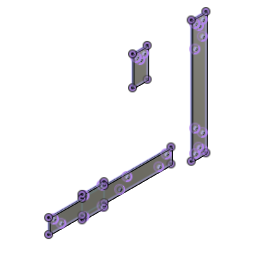
Chassis frame v4 (Autodesk Fusion 360 design; units mm, degrees)
Autodesk Fusion 360 part; units mm, degrees
sketch "Design sketch" plane through (0, 0, 0) normal (1, 0, 0) x (0, 1, 0)
  line L0 (125, 15) -> (-125, 15)
  line L1 (-125, 15) -> (-125, -15)
  line L2 (-125, -15) -> (125, -15)
  line L3 (125, -15) -> (125, 15)
  circle A0 centre (-100, -7.5) radius 1.75
  line L4 (196.3649, 218.9658) -> (166.3649, 218.9658)
  line L5 (166.3649, 218.9658) -> (166.3649, -31.0342)
  line L6 (196.3649, -31.0342) -> (196.3649, 218.9658)
  circle A1 centre (-115, 7.5) radius 1.75
  line L7 (166.3649, -31.0342) -> (196.3649, -31.0342)
  circle A2 centre (100, -7.5) radius 1.75
  circle A3 centre (115, 7.5) radius 1.75
  circle A4 centre (173.8649, 23.9658) radius 1.75
  circle A5 centre (188.8649, 8.9658) radius 1.75
  circle A6 centre (173.8649, 163.9658) radius 1.75
  circle A7 centre (188.8649, 178.9658) radius 1.75
  line L8 (-56.8073, -23.0185) -> (-11.8073, -23.0185)
  line L9 (-11.8073, -23.0185) -> (-11.8073, 21.9815)
  line L10 (-11.8073, 21.9815) -> (-56.8073, 21.9815)
  line L11 (-56.8073, 21.9815) -> (-56.8073, -23.0185)
  circle A8 centre (-52.8073, -19.0185) radius 1.75
  circle A9 centre (-52.8073, 17.9815) radius 1.75
  circle A10 centre (-15.8073, -19.0185) radius 1.75
  circle A11 centre (-15.8073, 17.9815) radius 1.75
  circle A12 centre (35, 7.5) radius 1.75
  circle A13 centre (20, -7.5) radius 1.75
  circle A14 centre (173.8649, -21.0342) radius 1.75
  circle A15 centre (188.8649, -21.0342) radius 1.75
  circle A16 centre (181.3649, -13.5342) radius 1.75
  circle A17 centre (173.8649, 208.9658) radius 1.75
  circle A18 centre (181.3649, 201.4658) radius 1.75
  circle A19 centre (188.8649, 208.9658) radius 1.75
  line L12 (46.3649, 218.9658) -> (76.3649, 218.9658)
  line L13 (76.3649, 218.9658) -> (76.3649, 158.9658)
  line L14 (76.3649, 158.9658) -> (46.3649, 158.9658)
  line L15 (46.3649, 158.9658) -> (46.3649, 218.9658)
  circle A20 centre (53.8649, 208.9658) radius 1.75
  circle A21 centre (61.3649, 201.4658) radius 1.75
  circle A22 centre (68.8649, 208.9658) radius 1.75
  point P0 (20, -7.5)
  dimension "d1" = 250
  dimension "d2" = 30
  dimension "d8" = 3.5
  dimension "d30" = 3.5
  dimension "d49" = 3.5
  dimension "d50" = 3.5
  dimension "d53" = 15
  dimension "d66" = 15
  dimension "d67" = 15
  dimension "d68" = 3.5
  dimension "d69" = 3.5
  dimension "d75" = 15
  dimension "d78" = 30
  dimension "d79" = 250
  dimension "d83" = 15
  dimension "d84" = 15
  dimension "d85" = 3.5
  dimension "d86" = 3.5
  dimension "d87" = 15
  dimension "d89" = 15
  dimension "d92" = 10
  dimension "d93" = 10
  dimension "d94" = 40
  dimension "d95" = 40
  dimension "d96" = 7.5
  dimension "d98" = 7.5
  dimension "d99" = 7.5
  dimension "d100" = 7.5
  dimension "d101" = 45
  dimension "d102" = 45
  dimension "d103" = 3.5
  dimension "d104" = 3.5
  dimension "d105" = 3.5
  dimension "d106" = 3.5
  dimension "d107" = 4
  dimension "d108" = 4
  dimension "d109" = 4
  dimension "d110" = 4
  dimension "d111" = 4
  dimension "d112" = 4
  dimension "d113" = 4
  dimension "d114" = 4
  dimension "d115" = 3.5
  dimension "d116" = 15
  dimension "d117" = 15
  dimension "d118" = 7.5
  dimension "d119" = 3.5
  dimension "d131" = 3.5
  dimension "d132" = 3.5
  dimension "d133" = 15
  dimension "d135" = 3.5
  dimension "d136" = 7.5
  dimension "d137" = 7.5
  dimension "d138" = 10
  dimension "d139" = 3.5
  dimension "d140" = 3.5
  dimension "d141" = 15
  dimension "d142" = 3.5
  dimension "d144" = 7.5
  dimension "d145" = 7.5
  dimension "d146" = 10
  dimension "d147" = 30
  dimension "d148" = 60
  dimension "d149" = 3.5
  dimension "d150" = 3.5
  dimension "d151" = 15
  dimension "d152" = 3.5
  dimension "d153" = 7.5
  dimension "d154" = 7.5
  dimension "d155" = 7.5
  dimension "d156" = 10
  constraint horizontal L0
  constraint perpendicular L0 L1
  constraint parallel L0 L2
  constraint parallel L1 L3
  constraint horizontal L4
  constraint perpendicular L4 L5
  constraint parallel L4 L7
  constraint parallel L5 L6
  constraint horizontal L8
  constraint vertical L9
  constraint horizontal L10
  constraint vertical L11
  constraint coincident P0 A13.centre
  constraint horizontal A14.centre A15.centre
  constraint horizontal A17.centre A19.centre
  constraint horizontal L12
  constraint vertical L13
  constraint horizontal L14
  constraint vertical L15
  constraint horizontal A20.centre A22.centre
  measures "d1" distance of L1.end L2.end
  measures "d2" distance of L0.end L1.end
  measures "d8" diameter of A0
  measures "d30" diameter of A1
  measures "d49" diameter of A2
  measures "d50" diameter of A3
  measures "d53" horizontal distance of A2.centre A3.centre
  measures "d66" vertical distance of A0.centre A1.centre
  measures "d67" horizontal distance of A0.centre A1.centre
  measures "d68" diameter of A4
  measures "d69" diameter of A5
  measures "d75" vertical distance of A2.centre A3.centre
  measures "d78" distance of L5.end L6.start
  measures "d79" distance of L4.start L6.start
  measures "d83" horizontal distance of A4.centre A5.centre
  measures "d84" vertical distance of A4.centre A5.centre
  measures "d85" diameter of A6
  measures "d86" diameter of A7
  measures "d87" horizontal distance of A6.centre A7.centre
  measures "d89" vertical distance of A6.centre A7.centre
  measures "d92" distance of L3 A3.centre
  measures "d93" distance of L1 A1.centre
  measures "d94" distance of L7 A5.centre
  measures "d95" distance of L4 A7.centre
  measures "d96" distance of L2 A2.centre
  measures "d98" distance of L5 A4.centre
  measures "d99" distance of L2 A0.centre
  measures "d100" distance of L5 A6.centre
  measures "d101" distance of L8.start L8.end
  measures "d102" distance of L8.start L10.end
  measures "d103" diameter of A8
  measures "d104" diameter of A9
  measures "d105" diameter of A10
  measures "d106" diameter of A11
  measures "d107" distance of L9 A10.centre
  measures "d108" distance of L8 A10.centre
  measures "d109" distance of L8 A8.centre
  measures "d110" distance of L11 A8.centre
  measures "d111" distance of L10 A9.centre
  measures "d112" distance of L11 A9.centre
  measures "d113" distance of L10 A11.centre
  measures "d114" distance of L9 A11.centre
  measures "d115" diameter of A12
  measures "d116" horizontal distance of P0 A12.centre
  measures "d117" vertical distance of P0 A12.centre
  measures "d118" distance of L2 P0
  measures "d119" diameter of A13
  measures "d131" diameter of A14
  measures "d132" diameter of A15
  measures "d133" horizontal distance of A14.centre A15.centre
  measures "d135" diameter of A16
  measures "d136" vertical distance of A14.centre A16.centre
  measures "d137" horizontal distance of A14.centre A16.centre
  measures "d138" distance of L7 A14.centre
  measures "d139" diameter of A17
  measures "d140" diameter of A19
  measures "d141" horizontal distance of A17.centre A19.centre
  measures "d142" diameter of A18
  measures "d144" horizontal distance of A18.centre A17.centre
  measures "d145" vertical distance of A18.centre A19.centre
  measures "d146" distance of L4 A19.centre
  measures "d147" distance of L12.start L12.end
  measures "d148" distance of L12.end L13.end
  measures "d149" diameter of A20
  measures "d150" diameter of A22
  measures "d151" horizontal distance of A20.centre A22.centre
  measures "d152" diameter of A21
  measures "d153" horizontal distance of A20.centre A21.centre
  measures "d154" vertical distance of A22.centre A21.centre
  measures "d155" distance of L15 A20.centre
  measures "d156" distance of L12 A20.centre
extrude "Extrude6" add sketch "Design sketch" along normal blind 3 makes body 1 at (0, -70.6452, -2.3357) makes body 2 at (0, 61.4084, 172.5507) makes body 3 at (0, 185.1196, 116.9837)
sketch "Sketch7" plane through (0, 0, 0) normal (1, 0, 0) x (0, 0, -1)
  circle A0 centre (-201.4658, 61.3649) radius 1.75
  circle A1 centre (-208.9658, 53.8649) radius 1.75
  circle A2 centre (-208.9658, 68.8649) radius 1.75
  line L0 (-158.9658, 46.3649) -> (-218.9658, 46.3649)
  line L1 (-218.9658, 46.3649) -> (-218.9658, 76.3649)
  line L2 (-218.9658, 76.3649) -> (-158.9658, 76.3649)
  line L3 (-158.9658, 76.3649) -> (-158.9658, 46.3649)
  circle A3 centre (-208.9658, 188.8649) radius 1.75
  circle A4 centre (-201.4658, 181.3649) radius 1.75
  circle A5 centre (-208.9658, 173.8649) radius 1.75
  circle A6 centre (13.5342, 181.3649) radius 1.75
  circle A7 centre (21.0342, 188.8649) radius 1.75
  circle A8 centre (21.0342, 173.8649) radius 1.75
  circle A9 centre (-178.9658, 188.8649) radius 1.75
  circle A10 centre (-8.9658, 188.8649) radius 1.75
  circle A11 centre (-163.9658, 173.8649) radius 1.75
  circle A12 centre (-23.9658, 173.8649) radius 1.75
  line L4 (-218.9658, 166.3649) -> (31.0342, 166.3649)
  line L5 (-218.9658, 196.3649) -> (-218.9658, 166.3649)
  line L6 (31.0342, 196.3649) -> (-218.9658, 196.3649)
  line L7 (31.0342, 166.3649) -> (31.0342, 196.3649)
  circle A13 centre (7.5, 20) radius 1.75
  circle A14 centre (-7.5, 35) radius 1.75
  circle A15 centre (-7.5, -115) radius 1.75
  circle A16 centre (-7.5, 115) radius 1.75
  circle A17 centre (7.5, 100) radius 1.75
  circle A18 centre (-17.9815, -52.8073) radius 1.75
  circle A19 centre (19.0185, -15.8073) radius 1.75
  circle A20 centre (7.5, -100) radius 1.75
  circle A21 centre (-17.9815, -15.8073) radius 1.75
  circle A22 centre (19.0185, -52.8073) radius 1.75
  line L8 (-21.9815, -11.8073) -> (-21.9815, -56.8073)
  line L9 (-15, -11.8073) -> (-21.9815, -11.8073)
  line L10 (-15, 125) -> (-15, -11.8073)
  line L11 (15, 125) -> (-15, 125)
  line L12 (15, -11.8073) -> (15, 125)
  line L13 (23.0185, -11.8073) -> (15, -11.8073)
  line L14 (23.0185, -56.8073) -> (23.0185, -11.8073)
  line L15 (15, -56.8073) -> (23.0185, -56.8073)
  line L16 (15, -125) -> (15, -56.8073)
  line L17 (-15, -125) -> (15, -125)
  line L18 (-15, -56.8073) -> (-15, -125)
  line L19 (-21.9815, -56.8073) -> (-15, -56.8073)
extrude "Extrude2" [suppressed]
equation "d1 = partLength"
equation "d2 = partWidth"
equation "partLength = 250 mm"
equation "partWidth = 30 mm"
equation "boltHole = 3.5 mm"
equation "d8 = boltHole"
equation "boltTriangleHeight = 7 mm"
equation "boltFromEdgesClose = 10 mm"
equation "boltGap = 15 mm"
equation "d30 = boltHole"
equation "boltFromEdgesFar = 40 mm"
equation "d49 = boltHole"
equation "d50 = boltHole"
equation "d53 = boltGap"
equation "d66 = boltGap"
equation "d67 = boltGap"
equation "d68 = boltHole"
equation "d69 = boltHole"
equation "d75 = boltGap"
equation "d78 = partWidth"
equation "d79 = partLength"
equation "d83 = boltGap"
equation "d84 = boltGap"
equation "d85 = boltHole"
equation "d86 = boltHole"
equation "d87 = boltGap"
equation "d89 = boltGap"
equation "d92 = boltFromEdgesClose"
equation "d93 = boltFromEdgesClose"
equation "d94 = boltFromEdgesFar"
equation "d95 = boltFromEdgesFar"
equation "d96 = ( partWidth - boltGap ) / 2"
equation "boltGapFromSide = ( partWidth - boltGap ) / 2"
equation "d98 = boltGapFromSide"
equation "d99 = boltGapFromSide"
equation "d100 = boltGapFromSide"
equation "d107 = ( ( 45 - 37 ) / 2 ) * 1 mm"
equation "d108 = ( ( 45 - 37 ) / 2 ) * 1 mm"
equation "d109 = ( ( 45 - 37 ) / 2 ) * 1 mm"
equation "d110 = ( ( 45 - 37 ) / 2 ) * 1 mm"
equation "d111 = ( ( 45 - 37 ) / 2 ) * 1 mm"
equation "d112 = ( ( 45 - 37 ) / 2 ) * 1 mm"
equation "d113 = ( ( 45 - 37 ) / 2 ) * 1 mm"
equation "d114 = ( ( 45 - 37 ) / 2 ) * 1 mm"
equation "d115 = boltHole"
equation "d116 = boltGap"
equation "d117 = boltGap"
equation "d118 = boltGapFromSide"
equation "d119 = boltHole"
equation "d131 = boltHole"
equation "d132 = boltHole"
equation "d133 = boltGap"
equation "d135 = boltHole"
equation "d136 = boltGap / 2"
equation "d137 = boltGap / 2"
equation "d139 = boltHole"
equation "d140 = boltHole"
equation "d141 = boltGap"
equation "d142 = boltHole"
equation "d144 = boltGap / 2"
equation "d145 = boltGap / 2"
equation "d147 = partWidth"
equation "d149 = boltHole"
equation "d150 = boltHole"
equation "d151 = boltGap"
equation "d152 = boltHole"
equation "d153 = boltGap / 2"
equation "d154 = boltGap / 2"
equation "d155 = boltGapFromSide"
